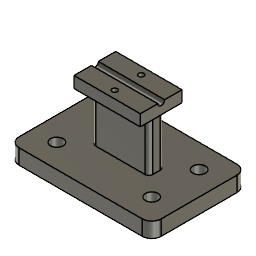
Fixed_Catheter_Clamp (Autodesk Fusion 360 design; units mm, degrees)
part number: 2026-08-12-14-12-58-001
part number: 2026-08-12-14-14-44-198
Autodesk Fusion 360 part; units mm, degrees
note: some values were not read from the file. Set by a fixed rule: which sketch regions a step uses.
sketch "草图1" plane through (0, 0, 0) normal (0, 0, 1) x (1, 0, 0)
  line L0 (37.5, -25) -> (-37.5, -25)
  line L1 (-37.5, -25) -> (-37.5, 25)
  line L2 (-37.5, 25) -> (37.5, 25)
  line L3 (37.5, 25) -> (37.5, -25)
  line L4 (37.5, -25) -> (-37.5, 25) construction
  line L5 (-37.5, -25) -> (37.5, 25) construction
  dimension "d34" = 75
  dimension "d35" = 50
  constraint horizontal L0
  constraint perpendicular L0 L1
  constraint parallel L0 L2
  constraint parallel L1 L3
  constraint coincident L4 origin
  constraint coincident L5 origin
  measures "d34" distance of L1.end L2.end
  measures "d35" distance of L0.start L2.end
extrude "拉伸1" add sketch "草图1" along normal blind 8
fillet "圆角1" radius 5 4 edges at (37.5, -25, 4) (-37.5, -25, 4) (37.5, 25, 4) (-37.5, 25, 4)
sketch "草图2" plane through (0, 0, 8) normal (0, 0, 1) x (-1, 0, 0)
  arc A0 (32.5, -25) -> (37.5, -20) centre (32.5, -20) ccw
  line L0 (37.5, -20) -> (37.5, 20)
  arc A1 (37.5, 20) -> (32.5, 25) centre (32.5, 20) ccw
  line L1 (32.5, 25) -> (-32.5, 25)
  arc A2 (-32.5, 25) -> (-37.5, 20) centre (-32.5, 20) ccw
  line L2 (-37.5, 20) -> (-37.5, -20)
  arc A3 (-37.5, -20) -> (-32.5, -25) centre (-32.5, -20) ccw
  line L3 (-32.5, -25) -> (32.5, -25)
  point P0 (-25, -12.5)
  dimension "d40" = 12.5
  dimension "d41" = 12.5
  measures "d40" distance of L3 P0
  measures "d41" distance of L2 P0
hole "孔1" at (25, 12.5, 8) direction (0, 0, -1) diameter 6.6 depth 25 tip angle 180
pattern_linear "R-阵列1" count 2 spacing 50 along (-1, 0, 0) count 2 spacing 25 along (0, -1, 0) of "孔1"
sketch "草图3" plane through (0, 0, 8) normal (0, 0, 1) x (-1, 0, 0)
  circle A0 centre (25, 12.5) radius 3.3
  circle A1 centre (-25, 12.5) radius 3.3
  circle A2 centre (25, -12.5) radius 3.3
  circle A3 centre (-25, -12.5) radius 3.3
  arc A4 (32.5, -25) -> (37.5, -20) centre (32.5, -20) ccw
  line L0 (37.5, -20) -> (37.5, 20)
  arc A5 (37.5, 20) -> (32.5, 25) centre (32.5, 20) ccw
  line L1 (32.5, 25) -> (-32.5, 25)
  arc A6 (-32.5, 25) -> (-37.5, 20) centre (-32.5, 20) ccw
  line L2 (-37.5, 20) -> (-37.5, -20)
  arc A7 (-37.5, -20) -> (-32.5, -25) centre (-32.5, -20) ccw
  line L3 (-32.5, -25) -> (32.5, -25)
  line L4 (15, -4) -> (-15, -4)
  line L5 (-15, -4) -> (-15, 4)
  line L6 (-15, 4) -> (15, 4)
  line L7 (15, 4) -> (15, -4)
  line L8 (15, -4) -> (-15, 4) construction
  line L9 (-15, -4) -> (15, 4) construction
  dimension "d49" = 30
  dimension "d50" = 8
  constraint horizontal L4
  constraint perpendicular L4 L5
  constraint parallel L4 L6
  constraint parallel L5 L7
  constraint coincident L8 origin
  constraint coincident L9 origin
  measures "d49" distance of L5.end L6.end
  measures "d50" distance of L4.start L6.end
extrude "拉伸2" add sketch "草图3" along normal blind 27.5 contours L4 L5 L6 L7
sketch "草图4" plane through (0, 0, 35.5) normal (0, 0, 1) x (-1, 0, 0)
  line L0 (15, 4) -> (-15, 4)
  line L1 (-15, 4) -> (-15, -4)
  line L2 (-15, -4) -> (15, -4)
  line L3 (15, -4) -> (15, 4)
  line L4 (17.5, -11) -> (-17.5, -11)
  line L5 (-17.5, -11) -> (-17.5, 11)
  line L6 (-17.5, 11) -> (17.5, 11)
  line L7 (17.5, 11) -> (17.5, -11)
  line L8 (17.5, -11) -> (-17.5, 11) construction
  line L9 (-17.5, -11) -> (17.5, 11) construction
  dimension "d53" = 35
  dimension "d54" = 22
  constraint horizontal L4
  constraint perpendicular L4 L5
  constraint parallel L4 L6
  constraint parallel L5 L7
  constraint coincident L8 origin
  constraint coincident L9 origin
  measures "d53" distance of L5.end L6.end
  measures "d54" distance of L4.start L6.end
extrude "拉伸3" add sketch "草图4" along normal blind 6 contours L0 L1 L2 L3 | L4 L5 L6 L7
sketch "草图5" plane through (0, 0, 0) normal (1, 0, 0) x (0, 1, 0)
  line L0 (11, 41.5) -> (-11, 41.5)
  line L1 (11, 35.5) -> (11, 41.5)
  line L2 (-11, 35.5) -> (-11, 41.5)
  circle A0 centre (0, 41.5) radius 1.8
  dimension "d57" = 3.6
  constraint midpoint L0 A0.centre
  measures "d57" diameter of A0
extrude "拉伸4" cut sketch "草图5" along normal blind 17.5 and the other way blind 17.5
sketch "草图6" plane through (0, 0, 41.5) normal (0, 0, 1) x (-1, 0, 0)
  line L0 (17.5, -1.8) -> (-17.5, -1.8)
  line L1 (-17.5, -1.8) -> (-17.5, -11)
  line L2 (-17.5, -11) -> (17.5, -11)
  line L3 (17.5, -11) -> (17.5, -1.8)
  point P0 (0, 7)
  point P1 (0, -7)
hole "孔2" at (0, -7, 41.5) at (0, 7, 41.5) direction (0, 0, -1) diameter 2.8 depth 10 tip angle 118
fillet "圆角2" radius 2 4 edges at (15, 4, 21.75) (-15, 4, 21.75) (15, -4, 21.75) (-15, -4, 21.75)
component "Fixed_Catheter_Clamp_Base" placed x (1, 0, 0) y (0, 1, 0) z (0, 0, 1) at (0, 0, 0)
equation "Rail_Support_Height = 8 mm" comment "【占位值】导入后必须改成实测值：实验台上表面到 MGN12 导轨底面的实际垂直距离；0 mm 不是设计值。"
equation "MGN12H_Combined_Height = 13 mm" comment "MGN12 导轨底面到 MGN12H 滑块顶面的组合高度"
equation "Pulley_Base_Thickness = 6 mm" comment "MGN12H 转接底座厚度"
equation "Wheel_Base_Clearance = 1.5 mm" comment "大导向轮底面与转接底座顶面的目标间隙"
equation "Pulley_Groove_Center_Height = 8 mm" comment "大导向轮底面到导管槽中心线的高度"
equation "Clamp_Center_Height = Rail_Support_Height + MGN12H_Combined_Height + Pulley_Base_Thickness + Wheel_Base_Clearance + Pulley_Groove_Center_Height" comment "固定夹导管中心距实验台面的高度；随 Rail_Support_Height 自动更新"
equation "Clamp_Base_Length = 75 mm" comment "桌面安装底板 X 方向长度"
equation "Clamp_Base_Width = 50 mm" comment "桌面安装底板 Y 方向宽度"
equation "Clamp_Base_Thickness = 8 mm" comment "桌面安装底板厚度"
equation "Clamp_Base_Corner_Radius = 5 mm" comment "底板四角圆角半径"
equation "Table_Hole_Pitch_X = 50 mm" comment "四个 M6 桌面安装孔 X 方向中心距"
equation "Table_Hole_Pitch_Y = 25 mm" comment "四个 M6 桌面安装孔 Y 方向中心距"
equation "M6_Clearance_Diameter = 6.6 mm" comment "M6 螺钉通孔直径"
equation "Column_Length = 30 mm" comment "中央立柱 X 方向长度"
equation "Column_Width = 20 mm" comment "中央立柱 Y 方向宽度"
equation "Lower_Jaw_Length = 35 mm" comment "下夹座 X 方向长度"
equation "Lower_Jaw_Width = 22 mm" comment "下夹座 Y 方向宽度"
equation "Lower_Jaw_Height = 6 mm" comment "下夹座高度"
equation "Column_Height = Clamp_Center_Height - Clamp_Base_Thickness - Lower_Jaw_Height" comment "中央立柱从底板顶面向上的高度；随 Rail_Support_Height 自动更新"
equation "Upper_Jaw_Length = 35 mm" comment "上夹盖 X 方向长度"
equation "Upper_Jaw_Width = 22 mm" comment "上夹盖 Y 方向宽度"
equation "Upper_Jaw_Height = 5 mm" comment "上夹盖高度"
equation "Catheter_Diameter = 2.4 mm" comment "弹簧导管外径"
equation "Ecoflex_Pad_Nominal_Thickness = 0.5 mm" comment "未来 Ecoflex 软垫名义厚度；本阶段只预留接口"
equation "Catheter_Assembly_Clearance = 0.2 mm" comment "导管与未来 Ecoflex 衬垫装配预留量"
equation "Clamp_Groove_Diameter = Catheter_Diameter + 2 * Ecoflex_Pad_Nominal_Thickness + Catheter_Assembly_Clearance" comment "硬质上下夹块导管槽直径；为未来 Ecoflex 衬垫预留"
equation "Clamp_M3_Offset_Y = 7 mm" comment "两枚 M3 螺钉相对夹块中心的 Y 向偏置"
equation "M3_Cap_Clearance_Diameter = 3.4 mm" comment "上夹盖 M3 通孔直径"
equation "M3_Lower_Pilot_Diameter = 2.8 mm" comment "下夹座 M3 导向孔直径"
equation "M3_Lower_Pilot_Depth = 5 mm" comment "下夹座 M3 导向孔深度"
equation "Column_Base_Fillet = 4 mm" comment "中央立柱与底板连接处圆角半径"
equation "Jaw_Column_Fillet = 2 mm" comment "下夹座与立柱连接处可选圆角半径"
equation "Edge_Fillet = 1 mm" comment "外部尖锐边缘小圆角半径"
equation "d34 = Clamp_Base_Length"
equation "d35 = Clamp_Base_Width"
equation "d36 = Clamp_Base_Thickness"
equation "d39 = Clamp_Base_Corner_Radius"
equation "d43 = M6_Clearance_Diameter"
equation "d49 = Column_Length"
equation "d50 = Column_Width / 2 - 2 mm"
equation "d51 = Column_Height + 5 mm"
equation "d53 = Lower_Jaw_Length"
equation "d54 = Lower_Jaw_Width"
equation "d55 = Lower_Jaw_Height"
equation "d57 = Clamp_Groove_Diameter"
equation "d62 = M3_Lower_Pilot_Depth + 5 mm"
equation "d63 = M3_Lower_Pilot_Diameter"
equation "d66 = Jaw_Column_Fillet"
